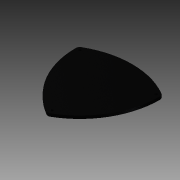
# Autodesk Inventor part: _BASALT BED
Saved by Autodesk Inventor 2013 (Build 170138000, 138)
## iProperties
Created: 2013-07-14
Part Number: _BASALT BED
Material: Generic
Document SubType Name: Modeling
Designer: employee
Density: 1 g/cm^3
Author: employee
Autodesk Inventor part; units mm, degrees
ref_plane "YZ Plane" through (0, 0, 0) normal (1, 0, 0) x (0, 1, 0)
ref_plane "XZ Plane" through (0, 0, 0) normal (0, 1, 0) x (-1, 0, 0)
ref_plane "XY Plane" through (0, 0, 0) normal (0, 0, 1) x (1, 0, 0)
sketch "Sketch1" plane through (0, 0, 0) normal (0, 0, 1) x (1, 0, 0)
  arc A0 (0, -144.3376) -> (125, 72.1688) centre (-125, 72.1688) ccw
  arc A1 (-125, 72.1688) -> (0, -144.3376) centre (125, 72.1688) ccw
  arc A2 (125, 72.1688) -> (-125, 72.1688) centre (0, -144.3376) ccw
  line L0 (-125, 72.1688) -> (0, 0) construction
  line L1 (0, 0) -> (125, 72.1688) construction
  line L2 (0, 0) -> (0, -144.3376) construction
  circle A3 centre (0, 0) radius 100
  arc A4 (-131.25, 82.9941) -> (-137.5, 72.1688) centre (-125, 72.1688) ccw
  arc A5 (137.5, 72.1688) -> (131.25, 82.9941) centre (125, 72.1688) ccw
  arc A6 (-6.25, -155.1629) -> (6.25, -155.1629) centre (0, -144.3376) ccw
  arc A7 (-137.5, 72.1688) -> (-6.25, -155.1629) centre (125, 72.1688) ccw
  arc A8 (131.25, 82.9941) -> (-131.25, 82.9941) centre (0, -144.3376) ccw
  arc A9 (6.25, -155.1629) -> (137.5, 72.1688) centre (-125, 72.1688) ccw
  line L3 (-100, 100) -> (100, 100)
  line L4 (100, 100) -> (100, -100)
  line L5 (100, -100) -> (-100, -100)
  line L6 (-100, -100) -> (-100, 100)
  point P0 (0, 0)
  point P1 (0, 0)
  dimension "d0" = 200
  dimension "d2" = 250
  dimension "d3" = 12.5
  constraints: 18 point on circle, 14 end point, 10 centre point, 10 coincident, 6 tangent, 2 equal length, 1 horizontal, 1 vertical, 9 other
  measures "d0" diameter of A3
  measures "d2" radius of A2
  measures "d3" radius of A5
extrude "Extrusion1" add sketch "Sketch1" along normal blind 9.525 contours A1 L5 A0 | A0 L5 A9 A6 A7 A1 | L5 A3 L4 A0 | A0 L4 A9 L5 | L5 A7 L6 A1 | A1 L6 A3 L5 | L4 A2 A0 | A0 A2 L4 A8 A5 A9 | A3 | L6 A7 A4 A8 A2 A1 | A1 A2 L6 | A3 L3 A2 L4 | L6 A2 L3 A3 | A2 L3 A8 L4 | L3 A2 | L6 A8 L3 A2 | A2 L3 A8
sketch "Sketch2" plane through (0, 0, 9.525) normal (0, 0, 1) x (1, 0, 0)
  arc A0 (131.25, 82.9941) -> (-131.25, 82.9941) centre (0, -144.3376) ccw projected
  arc A1 (-131.25, 82.9941) -> (-137.5, 72.1688) centre (-125, 72.1688) ccw projected
  arc A2 (-137.5, 72.1688) -> (-6.25, -155.1629) centre (125, 72.1688) ccw projected
  circle A3 centre (-125, 72.1688) radius 4.1
  circle A4 centre (125, 72.1688) radius 4.1
  circle A5 centre (0, -144.3376) radius 4.1
  point P0 (0, 0)
  dimension "d6" = 8.2
  constraints: 3 centre point, 3 coincident, 2 equal radius
  measures "d6" diameter of A3
extrude "Extrusion2" cut sketch "Sketch2" against normal through all
body "Solid1"
